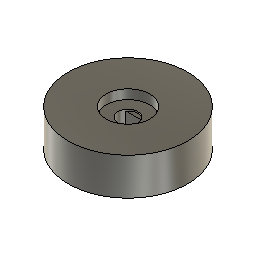
Monome Arc Clone - Knob (Autodesk Fusion 360 design; units mm, degrees)
Autodesk Fusion 360 part; units mm, degrees
cylinder "CylinderPrimitive1" add diameter 38.5 height 12 placed x (1, 0, 0) y (0, 1, 0) z (0, 0, 1) at (0, 0, 0) makes body 1
cylinder "CylinderPrimitive2" add diameter 6 height 10.5 placed x (1, 0, 0) y (0, 1, 0) z (0, 0, 1) at (25, 25, 0) separate body makes body 2
sketch "Sketch3" plane through (0, 0, 0) normal (1, 0, 0) x (0, 1, 0)
  line L0 (22, 10.5) -> (23.5, 10.5)
  line L1 (23.5, 10.5) -> (23.5, 3.5)
  line L2 (23.5, 3.5) -> (22, 3.5)
  line L3 (22, 3.5) -> (22, 10.5)
  dimension "d5" = 1.5
  dimension "d6" = 7
  constraint horizontal L0
  constraint vertical L1
  constraint horizontal L2
  constraint vertical L3
  measures "d5" distance of L0.start L0.end
  measures "d6" distance of L0.start L2.end
extrude "Extrude1" cut sketch "Sketch3" along normal blind 39 bodies 2
sketch "d-shaft" plane through (-21.35, 24.09, 0) normal (0, 0, 1) x (1, 0, 0)
  ellipse E0 centre (21.5358, -24.9167) end of major axis (22.2702, -28.6946) minor radius 3.3783 (21.3702, -21.0843) -> (19.8697, -21.4891) ccw
  line L0 (19.8697, -21.4891) -> (19.8697, -26.6805)
  spline S0 degree 3 poles (19.8697, -26.6805) (20.3114, -26.9365) (20.8229, -27.0853) (21.3702, -27.0853) (23.0274, -27.0853) (24.3707, -25.7419) (24.3707, -24.0848) (24.3707, -22.4277) (23.0274, -21.0843) (21.3702, -21.0843) knots 2 2 2 2 3 3 3 4 4 4 5 5 5 5
  spline S1 degree 3 poles (21.3707, -27.0853) (19.7139, -27.0853) (18.3707, -25.7422) (18.3707, -24.0853) knots 1 1 1 1 2 2 2 2
  spline S2 degree 3 poles (18.3707, -24.0853) (18.3707, -22.4285) (19.7139, -21.0853) (21.3707, -21.0853) knots 3 3 3 3 4 4 4 4
  spline S3 degree 3 poles (21.3707, -21.0853) (23.0276, -21.0853) (24.3707, -22.4285) (24.3707, -24.0853) knots 5 5 5 5 6 6 6 6
  spline S4 degree 3 poles (24.3707, -24.0853) (24.3707, -25.7422) (23.0276, -27.0853) (21.3707, -27.0853) knots 7 7 7 7 8 8 8 8
move_body "Move1" bodies 2 to x (1, 0, 0) y (0, 1, 0) z (0, 0, 1) at (-25, -25, 0)
combine "Combine1" operation cut target body 1 tool bodies 2
sketch "Sketch5" plane through (0, 0, 0) normal (0, 0, 1) x (1, 0, 0)
  circle A0 centre (0, 0) radius 5
  dimension "d9" = 10
  constraint coincident A0.centre origin
  measures "d9" diameter of A0
extrude "Extrude2" cut sketch "Sketch5" along normal blind 3 bodies 1
move_face "OffsetFaces1" offset -0.2 1 faces at (-2.7915, -1.0988, 5.5) on bodies 1
move_face "OffsetFaces2" offset -0.4 1 faces at (-0.9422, -1.5, 8.1667) on bodies 1
move_face "OffsetFaces3" offset -2 1 faces at (4.3673, -2.4345, 1.497) on bodies 1
move_body "Move2" bodies 1 to x (1, 0, 0) y (0, -1, 0) z (0, 0, -1) at (0, -38.5, 0)
